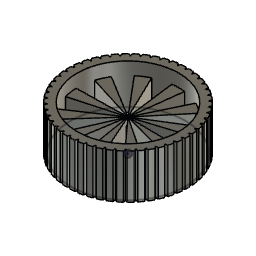
WallAce (Autodesk Fusion 360 archive; units mm, degrees)
design "Wheels"
part number: Configuration 2
Autodesk Fusion 360 part; units mm, degrees
sketch "Sketch1" plane through (0, 0, 0) normal (0, 0, 1) x (1, 0, 0)
  circle A0 centre (0, 0) radius 2.5
  circle A1 centre (0, 0) radius 40
  line L0 (0, 0) -> (4.8573, 39.704)
  line L1 (0, 0) -> (-4.3797, 39.7595)
  circle A2 centre (0, 0) radius 47
  dimension "d1" = 5
  dimension "d3" = 80
  dimension "d17" = 94
  constraint coincident A0.centre A1.centre
  constraint coincident A1 L0.end
  constraint coincident A1 L1.end
  measures "d1" diameter of A0
  measures "d3" diameter of A1
  measures "d17" diameter of A2
extrude "Extrude4" add sketch "Sketch1" along normal blind 20 makes body 1
sketch "Sketch6" plane through (0, 0, 0) normal (0, 0, -1) x (1, 0, 0)
  circle A0 centre (0, 0) radius 40
  circle A1 centre (0, 0) radius 47
  circle A2 centre (0, 0) radius 2.5
  dimension "d20" = 5
  constraint concentric A0 A2
  measures "d20" diameter of A2
sketch "Sketch7" plane through (0, 0, 0) normal (0, 0, -1) x (1, 0, 0)
sketch "Sketch8" plane through (0, 0, 0) normal (0, 0, -1) x (1, 0, 0)
sketch "Sketch9" plane through (0, 0, 0) normal (0, 0, -1) x (1, 0, 0)
sketch "Sketch10" plane through (0, 0, 0) normal (0, 0, -1) x (1, 0, 0)
extrude "Extrude5" add sketch "Sketch6" against normal blind 20 separate body contours A2 makes body 2
sketch "Sketch11" plane through (0, 0, 0) normal (0, 0, -1) x (1, 0, 0)
  circle A0 centre (0, 0) radius 40
  circle A1 centre (0, 0) radius 47
  line L0 (4.8914, -39.6998) -> (0, 0)
  line L1 (0, 0) -> (-5.0629, -39.6783)
  constraint coincident A0 L0.start
  constraint coincident A0.centre A1.centre
  constraint coincident A0 L1.end
extrude "Extrude6" add sketch "Sketch11" against normal blind 25 separate body contours A0 L0 L1 picked at (2.156, -26.5562) makes body 3
pattern_circular "C-Pattern2" count 11 over 360 about axis through (0, 0, 0) along (0, 0, 1) of bodies 3 makes body 4 at (-8.5703, 10.2141, 8.3333) makes body 5 at (-12.732, 3.9592, 8.3333) makes body 6 at (-12.8513, -3.5527, 8.3333) makes body 7 at (-8.8905, -9.9367, 8.3333) makes body 8 at (-2.1069, -13.1658, 8.3333) makes body 9 at (5.3455, -12.2149, 8.3333) makes body 10 at (11.1008, -7.3858, 8.3333) makes body 11 at (13.3317, -0.2118, 8.3333) makes body 12 at (11.3298, 7.0294, 8.3333) makes body 13 at (17.0522, 20.5021, 8.3333)
sketch "Sketch12" plane through (0, 0, 0) normal (0, 0, -1) x (1, 0, 0)
  circle A0 centre (0, 0) radius 2.5
  dimension "d27" = 5
  constraint coincident A0.centre origin
  measures "d27" diameter of A0
hole "Hole2" at (0, 0, 0) direction (0, 0, 1) diameter 5 depth 20 tip angle 180 bodies 2 3 4 5 6 7 8 9 10 11 12 13
extrude "Extrude7" add 1 faces at (6.276, 44.1314, 20) along direction (0, 0, 1) blind 15 on bodies 1 bodies 1 2
sketch "Sketch22" plane through (0, 0, 0) normal (0, 0, -1) x (1, 0, 0)
  circle A0 centre (0, 0) radius 40
  circle A1 centre (0, 0) radius 47
  circle A2 centre (0, 0) radius 45
  line L0 (-1.0373, 46.9886) -> (0, 45)
  line L1 (0, 45) -> (1.0373, 46.9886)
  dimension "d37" = 90
  constraint coincident A0.centre A1.centre
  constraint coincident A1 L0.start
  constraint coincident A2 L0.end
  constraint coincident A1 L1.end
  measures "d37" diameter of A2
sketch "Sketch28" plane through (0, 0, 0) normal (0, 0, -1) x (1, 0, 0)
  circle A0 centre (0, 0) radius 45
  dimension "d48" = 90
  constraint coincident A0.centre origin
  measures "d48" diameter of A0
sketch "Sketch29" plane through (0, 0, 0) normal (0, 0, -1) x (1, 0, 0)
  circle A0 centre (0, 0) radius 40
  circle A1 centre (0, 0) radius 47
  line L0 (-1.0142, 46.9891) -> (0, 45)
  line L1 (0, 45) -> (1.0142, 46.9891)
  constraint coincident A1 L0.start
  constraint coincident A1 L1.end
extrude "Extrude11" cut sketch "Sketch29" against normal blind 35 contours A1 L0 L1 picked at (0, 46.3325) bodies 1
pattern_circular "C-Pattern4" count 50 over 360 about axis through (0, 0, 0) along (0, 0, 1) of "Extrude11"
fillet "Fillet1" [rolled back] radius 15
sketch "Sketch23" plane through (0, 0, 0) normal (0, 0, -1) x (1, 0, 0)
  circle A0 centre (0, 0) radius 44
  dimension "d44" = 88
  constraint coincident A0.centre origin
  measures "d44" diameter of A0
sketch "Sketch24" plane through (0, 0, 0) normal (0, 0, -1) x (1, 0, 0)
sketch "Sketch25" plane through (0, 0, 0) normal (0, 0, -1) x (1, 0, 0)
sketch "Sketch26" plane through (0, 0, 0) normal (0, 0, -1) x (1, 0, 0)
  circle A0 centre (0, 0) radius 47
  line L0 (0, 44) -> (-8.8104, 46.1668)
  line L1 (0, 44) -> (-1.9328, 46.9602)
  dimension "d45" = 94
  constraint coincident A0.centre origin
  constraint coincident A0 L0.end
  constraint coincident A0 L1.end
  measures "d45" diameter of A0
extrude "Extrude10" [rolled back] along distance -15 taper angle 0
sketch "Sketch27" plane through (0, 0, 0) normal (0, 0, -1) x (1, 0, 0)
extrude "Extrude9" [suppressed]
pattern_circular "C-Pattern3" [suppressed]
extrude "Extrude1" [suppressed]
sketch "Sketch2" plane through (0, 0, 0) normal (0, 0, 1) x (1, 0, 0)
  circle A0 centre (0, 0) radius 2.5
  dimension "d6" = 5
  constraint coincident A0.centre origin
  measures "d6" diameter of A0
sketch "Sketch3" plane through (0, 0, 0) normal (0, 0, 1) x (1, 0, 0)
sketch "Sketch4" plane through (0, 0, 0) normal (0, 0, -1) x (1, 0, 0)
  circle A0 centre (0, 0) radius 40
  circle A1 centre (0, 0) radius 49
  line L0 (5.0094, -39.6851) -> (0, 0)
  line L1 (0, 0) -> (-5.0094, -39.6851)
  constraint coincident A0 L0.start
  constraint coincident A0.centre A1.centre
  constraint coincident A0 L1.end
extrude "Extrude2" [suppressed]
pattern_circular "C-Pattern1" [suppressed]
sketch "Sketch5" plane through (0, 0, 0) normal (0, 0, 1) x (1, 0, 0)
  circle A0 centre (0, 0) radius 2.5
  dimension "d11" = 5
  constraint coincident A0.centre origin
  measures "d11" diameter of A0
hole "Hole1" [suppressed]
extrude "Extrude3" [suppressed]

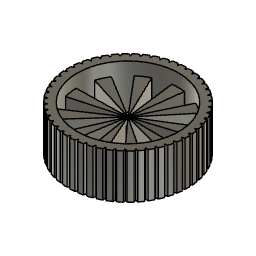
design "small wh"
part number: Configuration 2
Autodesk Fusion 360 part; units mm, degrees
sketch "Sketch1" plane through (0, 0, 0) normal (0, 0, 1) x (1, 0, 0)
  circle A0 centre (0, 0) radius 2.5
  circle A1 centre (0, 0) radius 40
  line L0 (0, 0) -> (4.8573, 39.704)
  line L1 (0, 0) -> (-4.3797, 39.7595)
  circle A2 centre (0, 0) radius 47
  dimension "d1" = 5
  dimension "d3" = 80
  dimension "d17" = 94
  constraint coincident A0.centre A1.centre
  constraint coincident A1 L0.end
  constraint coincident A1 L1.end
  measures "d1" diameter of A0
  measures "d3" diameter of A1
  measures "d17" diameter of A2
extrude "Extrude4" add sketch "Sketch1" along normal blind 20 makes body 1
sketch "Sketch6" plane through (0, 0, 0) normal (0, 0, -1) x (1, 0, 0)
  circle A0 centre (0, 0) radius 40
  circle A1 centre (0, 0) radius 47
  circle A2 centre (0, 0) radius 2.5
  dimension "d20" = 5
  constraint concentric A0 A2
  measures "d20" diameter of A2
sketch "Sketch7" plane through (0, 0, 0) normal (0, 0, -1) x (1, 0, 0)
sketch "Sketch8" plane through (0, 0, 0) normal (0, 0, -1) x (1, 0, 0)
sketch "Sketch9" plane through (0, 0, 0) normal (0, 0, -1) x (1, 0, 0)
sketch "Sketch10" plane through (0, 0, 0) normal (0, 0, -1) x (1, 0, 0)
extrude "Extrude5" add sketch "Sketch6" against normal blind 20 separate body contours A2 makes body 2
sketch "Sketch11" plane through (0, 0, 0) normal (0, 0, -1) x (1, 0, 0)
  circle A0 centre (0, 0) radius 40
  circle A1 centre (0, 0) radius 47
  line L0 (4.8914, -39.6998) -> (0, 0)
  line L1 (0, 0) -> (-5.0629, -39.6783)
  constraint coincident A0 L0.start
  constraint coincident A0.centre A1.centre
  constraint coincident A0 L1.end
extrude "Extrude6" add sketch "Sketch11" against normal blind 25 separate body contours A0 L0 L1 picked at (2.156, -26.5562) makes body 3
pattern_circular "C-Pattern2" count 11 over 360 about axis through (0, 0, 0) along (0, 0, 1) of bodies 3 makes body 4 at (-8.5703, 10.2141, 8.3333) makes body 5 at (-12.732, 3.9592, 8.3333) makes body 6 at (-12.8513, -3.5527, 8.3333) makes body 7 at (-8.8905, -9.9367, 8.3333) makes body 8 at (-2.1069, -13.1658, 8.3333) makes body 9 at (5.3455, -12.2149, 8.3333) makes body 10 at (11.1008, -7.3858, 8.3333) makes body 11 at (13.3317, -0.2118, 8.3333) makes body 12 at (11.3298, 7.0294, 8.3333) makes body 13 at (17.0522, 20.5021, 8.3333)
sketch "Sketch12" plane through (0, 0, 0) normal (0, 0, -1) x (1, 0, 0)
  circle A0 centre (0, 0) radius 2.5
  dimension "d27" = 5
  constraint coincident A0.centre origin
  measures "d27" diameter of A0
hole "Hole2" at (0, 0, 0) direction (0, 0, 1) diameter 5 depth 20 tip angle 180 bodies 2 3 4 5 6 7 8 9 10 11 12 13
extrude "Extrude7" add 1 faces at (6.276, 44.1314, 20) along direction (0, 0, 1) blind 15 on bodies 1 bodies 1 2
sketch "Sketch22" plane through (0, 0, 0) normal (0, 0, -1) x (1, 0, 0)
  circle A0 centre (0, 0) radius 40
  circle A1 centre (0, 0) radius 47
  circle A2 centre (0, 0) radius 45
  line L0 (-1.0373, 46.9886) -> (0, 45)
  line L1 (0, 45) -> (1.0373, 46.9886)
  dimension "d37" = 90
  constraint coincident A0.centre A1.centre
  constraint coincident A1 L0.start
  constraint coincident A2 L0.end
  constraint coincident A1 L1.end
  measures "d37" diameter of A2
sketch "Sketch28" plane through (0, 0, 0) normal (0, 0, -1) x (1, 0, 0)
sketch "Sketch29" plane through (0, 0, 0) normal (0, 0, -1) x (1, 0, 0)
  circle A0 centre (0, 0) radius 40
  circle A1 centre (0, 0) radius 47
  line L0 (-1.0142, 46.9891) -> (0, 45)
  line L1 (0, 45) -> (1.0142, 46.9891)
  constraint coincident A1 L0.start
  constraint coincident A1 L1.end
extrude "Extrude11" cut sketch "Sketch29" against normal blind 35 contours A1 L0 L1 picked at (0, 46.3325) bodies 1
pattern_circular "C-Pattern4" count 50 over 360 about axis through (0, 0, 0) along (0, 0, 1) of "Extrude11"
scale "Scale1" factor 1 about (-40, 0, 35) bodies 1 10
scale "Scale2" factor 0.375815 about (-40, 0, 35) bodies 12 9 3 6 11 13 7 10 8 1 4 5
fillet "Fillet1" [suppressed]
sketch "Sketch23" plane through (0, 0, 0) normal (0, 0, -1) x (1, 0, 0)
  circle A0 centre (0, 0) radius 44
  dimension "d44" = 88
  constraint coincident A0.centre origin
  measures "d44" diameter of A0
sketch "Sketch24" plane through (0, 0, 0) normal (0, 0, -1) x (1, 0, 0)
sketch "Sketch25" plane through (0, 0, 0) normal (0, 0, -1) x (1, 0, 0)
sketch "Sketch26" plane through (0, 0, 0) normal (0, 0, -1) x (1, 0, 0)
  circle A0 centre (0, 0) radius 47
  line L0 (0, 44) -> (-8.8104, 46.1668)
  line L1 (0, 44) -> (-1.9328, 46.9602)
  dimension "d45" = 94
  constraint coincident A0.centre origin
  constraint coincident A0 L0.end
  constraint coincident A0 L1.end
  measures "d45" diameter of A0
extrude "Extrude10" [suppressed]
sketch "Sketch27" plane through (0, 0, 0) normal (0, 0, -1) x (1, 0, 0)
extrude "Extrude9" [suppressed]
pattern_circular "C-Pattern3" [suppressed]
extrude "Extrude1" [suppressed]
sketch "Sketch2" plane through (0, 0, 0) normal (0, 0, 1) x (1, 0, 0)
  circle A0 centre (0, 0) radius 2.5
  dimension "d6" = 5
  constraint coincident A0.centre origin
  measures "d6" diameter of A0
sketch "Sketch3" plane through (0, 0, 0) normal (0, 0, 1) x (1, 0, 0)
sketch "Sketch4" plane through (0, 0, 0) normal (0, 0, -1) x (1, 0, 0)
  circle A0 centre (0, 0) radius 40
  circle A1 centre (0, 0) radius 49
  line L0 (5.0094, -39.6851) -> (0, 0)
  line L1 (0, 0) -> (-5.0094, -39.6851)
  constraint coincident A0 L0.start
  constraint coincident A0.centre A1.centre
  constraint coincident A0 L1.end
extrude "Extrude2" [suppressed]
pattern_circular "C-Pattern1" [suppressed]
sketch "Sketch5" plane through (0, 0, 0) normal (0, 0, 1) x (1, 0, 0)
  circle A0 centre (0, 0) radius 2.5
  dimension "d11" = 5
  constraint coincident A0.centre origin
  measures "d11" diameter of A0
hole "Hole1" [suppressed]
extrude "Extrude3" [suppressed]

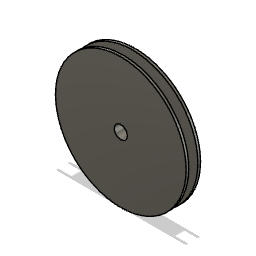
design "pully p1"
Autodesk Fusion 360 part; units mm, degrees
cylinder "CylinderPrimitive1" add diameter 40 height 3.5 placed x (1, 0, 0) y (0, 1, 0) z (0, 0, 1) at (0, 0, 0)
cylinder "CylinderPrimitive2" add diameter 50 height 1 placed x (1, 0, 0) y (0, 1, 0) z (0, 0, 1) at (0, 0, 3.5)
cylinder "CylinderPrimitive3" add diameter 50 height 1 placed x (0, 1, 0) y (1, 0, 0) z (0, 0, -1) at (0, 0, 0)
hole "Hole1" at (0, 0, -1) direction (0, 0, 1) diameter 5 depth 55 counterbore diameter 7 counterbore depth 0.01
